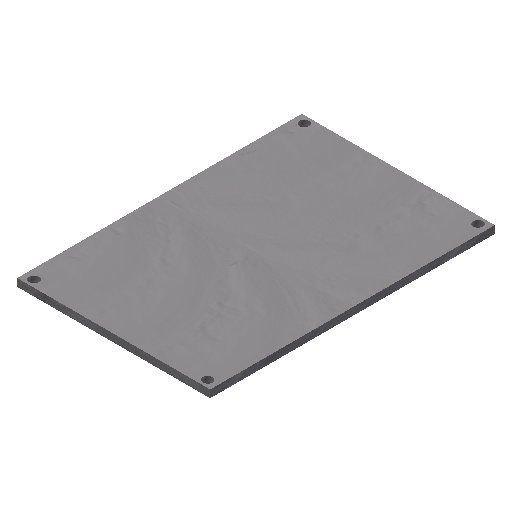
# Autodesk Inventor part: pcb sola
Saved by Autodesk Inventor 2025.2 (Build 292293000, 293)
## iProperties
Created: 2025-10-17
Part Number: pcb sola
Material: Steel, Mild, Welded
Document SubType Name: Modeling
Designer: Ricardo
Density: 7.85 g/cm^3
Appearance: Weld - Steel Mild
Author: Ricardo
Autodesk Inventor part; units mm, degrees
ref_plane "YZ Plane" through (0, 0, 0) normal (1, 0, 0) x (0, 1, 0)
ref_plane "XZ Plane" through (0, 0, 0) normal (0, 1, 0) x (-1, 0, 0)
ref_plane "XY Plane" through (0, 0, 0) normal (0, 0, 1) x (1, 0, 0)
sketch "Sketch1" plane through (0, 0, 0) normal (0, 1, 0) x (-1, 0, 0)
  line L0 (0, 0) -> (40, 0)
  line L1 (40, 0) -> (40, -59)
  line L2 (40, -59) -> (0, -59)
  line L3 (0, -59) -> (0, 0)
  dimension "d0" = 40
  dimension "d1" = 59
  constraints: 8 end point, 2 parallel, 1 horizontal, 1 perpendicular
  measures "d0" distance of L1.end L2.end
  measures "d1" distance of L0.end L1.end
extrude "Extrusion1" add sketch "Sketch1" along normal blind 1.57
sketch "Sketch2" plane through (0, 1.57, 0) normal (0, 1, 0) x (1, 0, 0)
  circle A0 centre (-38, 1.5) radius 1
  line L0 (-40, 59) -> (-40, 0) projected
  line L1 (-40, 0) -> (0, 0) projected
  line L2 (0, 59) -> (-40, 59) projected
  line L3 (-40, 59) -> (-40, 0) projected
  line L4 (-40, 0) -> (0, 0) projected
  line L5 (0, 0) -> (0, 59) projected
  line L6 (0, 0) -> (0, 59) projected
  line L7 (0, 59) -> (-40, 59) projected
  line L8 (0, 29.5) -> (-40, 29.5)
  line L9 (-20, 0) -> (-20, 59)
  circle A1 centre (-38, 57.5) radius 1
  circle A2 centre (-2, 1.5) radius 1
  circle A3 centre (-2, 57.5) radius 1
  dimension "d4" = 2
  dimension "d5" = 2
  dimension "d6" = 1.5
  constraints: 4 centre point, 4 end point, 4 midpoint, 3 symmetric about line, 3 other
  measures "d4" diameter of A0
  measures "d5" distance from line of L0 A0.centre
  measures "d6" distance from line of L1 A0.centre
extrude "Extrusion2" cut sketch "Sketch2" against normal blind 2 contours A0 | A1 | A2 | A3
equation "\"d7\" = d4"
body "Solid1"
